Autodesk Inventor part; units mm, degrees
(part 4 of 4)
sketch "Sketch8" plane through (0, 0, 5) normal (0, 0, 1) x (1, 0, 0)
  line L0 (-35.5504, 47.4568) -> (35.8971, 47.4568) construction
  line L1 (35.8971, 47.4568) -> (35.8971, 30.428) construction
  line L2 (35.8971, 30.428) -> (-35.5504, 30.428) construction
  line L3 (-35.5504, 30.428) -> (-35.5504, 47.4568) construction
  line L4 (0.1734, 55.1961) -> (0.1734, 17.6773) construction
  line L5 (0, -39.5) -> (0, 79.5) construction
  spline S0 degree 2 poles (-22.5428, 39.6572) (-23.4481, 39.1897) (-24.7914, 39.1897) knots 0 0 0 1 1 1
  spline S1 degree 2 poles (-24.7914, 39.1897) (-26.5353, 39.1897) (-28.6281, 41.3863) (-28.6281, 43.1748) knots 0 0 0 1 2 2 2
  spline S2 degree 2 poles (-28.6281, 43.1748) (-28.6281, 45.0895) (-26.2682, 47.4568) (-24.4648, 47.4568) knots 0 0 0 1 2 2 2
  spline S3 degree 2 poles (-24.4648, 47.4568) (-23.3071, 47.4568) (-22.5428, 47.1303) knots 0 0 0 1 1 1
  line L6 (-22.5428, 47.1303) -> (-22.5428, 45.8093)
  spline S4 degree 2 poles (-22.5428, 45.8093) (-23.3517, 46.2917) (-24.3313, 46.2917) knots 0 0 0 1 1 1
  spline S5 degree 2 poles (-24.3313, 46.2917) (-25.63, 46.2917) (-27.2403, 44.6294) (-27.2403, 43.2416) knots 0 0 0 1 2 2 2
  spline S6 degree 2 poles (-27.2403, 43.2416) (-27.2403, 41.9132) (-25.7339, 40.3474) (-24.5094, 40.3474) knots 0 0 0 1 2 2 2
  spline S7 degree 2 poles (-24.5094, 40.3474) (-23.3739, 40.3474) (-22.5428, 40.8817) knots 0 0 0 1 1 1
  line L7 (-22.5428, 40.8817) -> (-22.5428, 39.6572)
  line L8 (-14.6021, 39.3232) -> (-15.9305, 39.3232)
  line L9 (-15.9305, 39.3232) -> (-15.9305, 42.7963)
  line L10 (-15.9305, 42.7963) -> (-19.7005, 42.7963)
  line L11 (-19.7005, 42.7963) -> (-19.7005, 39.3232)
  line L12 (-19.7005, 39.3232) -> (-21.0288, 39.3232)
  line L13 (-21.0288, 39.3232) -> (-21.0288, 47.3232)
  line L14 (-21.0288, 47.3232) -> (-19.7005, 47.3232)
  line L15 (-19.7005, 47.3232) -> (-19.7005, 43.9615)
  line L16 (-19.7005, 43.9615) -> (-15.9305, 43.9615)
  line L17 (-15.9305, 43.9615) -> (-15.9305, 47.3232)
  line L18 (-15.9305, 47.3232) -> (-14.6021, 47.3232)
  line L19 (-14.6021, 47.3232) -> (-14.6021, 39.3232)
  line L20 (-6.053, 39.3232) -> (-7.5075, 39.3232)
  line L21 (-7.5075, 39.3232) -> (-8.2274, 41.3566)
  line L22 (-8.2274, 41.3566) -> (-11.3739, 41.3566)
  line L23 (-11.3739, 41.3566) -> (-12.0715, 39.3232)
  line L24 (-12.0715, 39.3232) -> (-13.5186, 39.3232)
  line L25 (-13.5186, 39.3232) -> (-10.5205, 47.3232)
  line L26 (-10.5205, 47.3232) -> (-9.0288, 47.3232)
  line L27 (-9.0288, 47.3232) -> (-6.053, 39.3232)
  line L28 (-8.5836, 42.4401) -> (-9.6893, 45.6312)
  spline S8 degree 2 poles (-9.6893, 45.6312) (-9.7413, 45.7871) (-9.8006, 46.1359) knots 0 0 0 1 1 1
  line L29 (-9.8006, 46.1359) -> (-9.8229, 46.1359)
  spline S9 degree 2 poles (-9.8229, 46.1359) (-9.8674, 45.8168) (-9.9342, 45.6312) knots 0 0 0 1 1 1
  line L30 (-9.9342, 45.6312) -> (-11.0326, 42.4401)
  line L31 (-11.0326, 42.4401) -> (-8.5836, 42.4401)
  line L32 (-0.5242, 39.3232) -> (-4.9546, 39.3232)
  line L33 (-4.9546, 39.3232) -> (-4.9546, 47.3232)
  line L34 (-4.9546, 47.3232) -> (-3.6262, 47.3232)
  line L35 (-3.6262, 47.3232) -> (-3.6262, 40.4438)
  line L36 (-3.6262, 40.4438) -> (-0.5242, 40.4438)
  line L37 (-0.5242, 40.4438) -> (-0.5242, 39.3232)
  line L38 (9.2272, 39.3232) -> (7.9136, 39.3232)
  line L39 (7.9136, 39.3232) -> (7.9136, 44.5032)
  spline S10 degree 2 poles (7.9136, 44.5032) (7.9136, 45.134) (7.9879, 46.0542) knots 0 0 0 1 1 1
  line L40 (7.9879, 46.0542) -> (7.9656, 46.0542)
  spline S11 degree 2 poles (7.9656, 46.0542) (7.8469, 45.5348) (7.7504, 45.3047) knots 0 0 0 1 1 1
  line L41 (7.7504, 45.3047) -> (5.3608, 39.3232)
  line L42 (5.3608, 39.3232) -> (4.448, 39.3232)
  line L43 (4.448, 39.3232) -> (2.0509, 45.2602)
  spline S12 degree 2 poles (2.0509, 45.2602) (1.9545, 45.5199) (1.8431, 46.0542) knots 0 0 0 1 1 1
  line L44 (1.8431, 46.0542) -> (1.8209, 46.0542)
  spline S13 degree 2 poles (1.8209, 46.0542) (1.8654, 45.5793) (1.8654, 44.4884) knots 0 0 0 1 1 1
  line L45 (1.8654, 44.4884) -> (1.8654, 39.3232)
  line L46 (1.8654, 39.3232) -> (0.6335, 39.3232)
  line L47 (0.6335, 39.3232) -> (0.6335, 47.3232)
  line L48 (0.6335, 47.3232) -> (2.5036, 47.3232)
  line L49 (2.5036, 47.3232) -> (4.6038, 41.9949)
  spline S14 degree 2 poles (4.6038, 41.9949) (4.8487, 41.3789) (4.9229, 41.0821) knots 0 0 0 1 1 1
  line L50 (4.9229, 41.0821) -> (4.9452, 41.0821)
  spline S15 degree 2 poles (4.9452, 41.0821) (5.153, 41.7129) (5.2791, 42.0171) knots 0 0 0 1 1 1
  line L51 (5.2791, 42.0171) -> (7.4238, 47.3232)
  line L52 (7.4238, 47.3232) -> (9.2272, 47.3232)
  line L53 (9.2272, 47.3232) -> (9.2272, 39.3232)
  line L54 (15.6836, 39.3232) -> (11.1938, 39.3232)
  line L55 (11.1938, 39.3232) -> (11.1938, 47.3232)
  line L56 (11.1938, 47.3232) -> (15.5055, 47.3232)
  line L57 (15.5055, 47.3232) -> (15.5055, 46.1952)
  line L58 (15.5055, 46.1952) -> (12.5222, 46.1952)
  line L59 (12.5222, 46.1952) -> (12.5222, 43.9318)
  line L60 (12.5222, 43.9318) -> (15.2754, 43.9318)
  line L61 (15.2754, 43.9318) -> (15.2754, 42.8112)
  line L62 (15.2754, 42.8112) -> (12.5222, 42.8112)
  line L63 (12.5222, 42.8112) -> (12.5222, 40.4438)
  line L64 (12.5222, 40.4438) -> (15.6836, 40.4438)
  line L65 (15.6836, 40.4438) -> (15.6836, 39.3232)
  line L66 (23.2903, 39.3232) -> (21.7392, 39.3232)
  line L67 (21.7392, 39.3232) -> (20.4628, 41.468)
  spline S16 degree 2 poles (20.4628, 41.468) (20.2921, 41.7648) (19.9582, 42.1804) (19.6168, 42.4476) (19.2161, 42.5737) (18.9712, 42.5737) knots 0 0 0 1 2 3 4 4 4
  line L68 (18.9712, 42.5737) -> (18.4294, 42.5737)
  line L69 (18.4294, 42.5737) -> (18.4294, 39.3232)
  line L70 (18.4294, 39.3232) -> (17.1084, 39.3232)
  line L71 (17.1084, 39.3232) -> (17.1084, 47.3232)
  line L72 (17.1084, 47.3232) -> (19.743, 47.3232)
  spline S17 degree 2 poles (19.743, 47.3232) (20.307, 47.3232) (21.2569, 47.0561) (21.9619, 46.5143) (22.3552, 45.7054) (22.3552, 45.1637) knots 0 0 0 1 2 3 4 4 4
  spline S18 degree 2 poles (22.3552, 45.1637) (22.3552, 44.7407) (22.1029, 44.0357) (21.6428, 43.4791) (20.9897, 43.0932) (20.5815, 42.9893) knots 0 0 0 1 2 3 4 4 4
  line L73 (20.5815, 42.9893) -> (20.5815, 42.967)
  spline S19 degree 2 poles (20.5815, 42.967) (20.7968, 42.8409) (21.1233, 42.544) (21.4127, 42.2323) (21.6947, 41.839) (21.8728, 41.5719) knots 0 0 0 1 2 3 4 4 4
  line L74 (21.8728, 41.5719) -> (23.2903, 39.3232)
  line L75 (18.4294, 46.2472) -> (18.4294, 43.6498)
  line L76 (18.4294, 43.6498) -> (19.5352, 43.6498)
  spline S20 degree 2 poles (19.5352, 43.6498) (19.8469, 43.6498) (20.3589, 43.8427) (20.7448, 44.1989) (20.9526, 44.711) (20.9526, 45.0301) knots 0 0 0 1 2 3 4 4 4
  spline S21 degree 2 poles (20.9526, 45.0301) (20.9526, 45.6015) (20.2253, 46.2472) (19.55, 46.2472) knots 0 0 0 1 2 2 2
  line L77 (19.55, 46.2472) -> (18.4294, 46.2472)
  line L78 (23.8543, 39.6424) -> (23.8543, 41.0078)
  spline S22 degree 2 poles (23.8543, 41.0078) (24.0398, 40.8372) (24.5519, 40.57) (25.1159, 40.3919) (25.6873, 40.288) (25.9248, 40.288) knots 0 0 0 1 2 3 4 4 4
  spline S23 degree 2 poles (25.9248, 40.288) (26.7634, 40.288) (27.5871, 40.8446) (27.5871, 41.3789) knots 0 0 0 1 2 2 2
  spline S24 degree 2 poles (27.5871, 41.3789) (27.5871, 41.6609) (27.3125, 42.0765) (26.8227, 42.4253) (26.1548, 42.7444) (25.7764, 42.9151) knots 0 0 0 1 2 3 4 4 4
  spline S25 degree 2 poles (25.7764, 42.9151) (25.3682, 43.1303) (24.6706, 43.583) (24.1511, 44.1173) (23.8543, 44.8001) (23.8543, 45.2602) knots 0 0 0 1 2 3 4 4 4
  spline S26 degree 2 poles (23.8543, 45.2602) (23.8543, 45.8242) (24.3589, 46.6553) (25.1901, 47.1971) (26.2513, 47.4568) (26.8079, 47.4568) knots 0 0 0 1 2 3 4 4 4
  spline S27 degree 2 poles (26.8079, 47.4568) (28.0621, 47.4568) (28.6335, 47.1748) knots 0 0 0 1 1 1
  line L79 (28.6335, 47.1748) -> (28.6335, 45.8613)
  spline S28 degree 2 poles (28.6335, 45.8613) (27.9507, 46.3511) (26.8821, 46.3511) knots 0 0 0 1 1 1
  spline S29 degree 2 poles (26.8821, 46.3511) (26.5853, 46.3511) (25.999, 46.2398) (25.5389, 45.98) (25.2494, 45.5793) (25.2494, 45.2973) knots 0 0 0 1 2 3 4 4 4
  spline S30 degree 2 poles (25.2494, 45.2973) (25.2494, 45.0301) (25.4721, 44.6368) (25.9025, 44.3177) (26.5185, 44.006) (26.9266, 43.8279) knots 0 0 0 1 2 3 4 4 4
  spline S31 degree 2 poles (26.9266, 43.8279) (27.3422, 43.6127) (28.0843, 43.1303) (28.6483, 42.5514) (28.9823, 41.8464) (28.9823, 41.3937) knots 0 0 0 1 2 3 4 4 4
  spline S32 degree 2 poles (28.9823, 41.3937) (28.9823, 40.7852) (28.4925, 39.9466) (27.6613, 39.4271) (26.5778, 39.1897) (25.9693, 39.1897) knots 0 0 0 1 2 3 4 4 4
  spline S33 degree 2 poles (25.9693, 39.1897) (25.7689, 39.1897) (25.1827, 39.249) (24.5741, 39.3678) (24.025, 39.5385) (23.8543, 39.6424) knots 0 0 0 1 2 3 4 4 4
  line L80 (-23.3851, 31.9735) -> (-26.257, 23.9735)
  line L81 (-26.257, 23.9735) -> (-27.7413, 23.9735)
  line L82 (-27.7413, 23.9735) -> (-30.5613, 31.9735)
  line L83 (-30.5613, 31.9735) -> (-29.1142, 31.9735)
  line L84 (-29.1142, 31.9735) -> (-27.1402, 25.903)
  spline S34 degree 2 poles (-27.1402, 25.903) (-27.0437, 25.6136) (-26.9917, 25.2277) knots 0 0 0 1 1 1
  line L85 (-26.9917, 25.2277) -> (-26.9695, 25.2277)
  spline S35 degree 2 poles (-26.9695, 25.2277) (-26.9324, 25.5468) (-26.8062, 25.9179) knots 0 0 0 1 1 1
  line L86 (-26.8062, 25.9179) -> (-24.7877, 31.9735)
  line L87 (-24.7877, 31.9735) -> (-23.3851, 31.9735)
  line L88 (-17.834, 23.9735) -> (-22.3238, 23.9735)
  line L89 (-22.3238, 23.9735) -> (-22.3238, 31.9735)
  line L90 (-22.3238, 31.9735) -> (-18.0121, 31.9735)
  line L91 (-18.0121, 31.9735) -> (-18.0121, 30.8455)
  line L92 (-18.0121, 30.8455) -> (-20.9954, 30.8455)
  line L93 (-20.9954, 30.8455) -> (-20.9954, 28.582)
  line L94 (-20.9954, 28.582) -> (-18.2422, 28.582)
  line L95 (-18.2422, 28.582) -> (-18.2422, 27.4614)
  line L96 (-18.2422, 27.4614) -> (-20.9954, 27.4614)
  line L97 (-20.9954, 27.4614) -> (-20.9954, 25.0941)
  line L98 (-20.9954, 25.0941) -> (-17.834, 25.0941)
  line L99 (-17.834, 25.0941) -> (-17.834, 23.9735)
  line L100 (-10.2274, 23.9735) -> (-11.7784, 23.9735)
  line L101 (-11.7784, 23.9735) -> (-13.0548, 26.1182)
  spline S36 degree 2 poles (-13.0548, 26.1182) (-13.2255, 26.4151) (-13.5595, 26.8307) (-13.9008, 27.0978) (-14.3016, 27.224) (-14.5465, 27.224) knots 0 0 0 1 2 3 4 4 4
  line L102 (-14.5465, 27.224) -> (-15.0882, 27.224)
  line L103 (-15.0882, 27.224) -> (-15.0882, 23.9735)
  line L104 (-15.0882, 23.9735) -> (-16.4092, 23.9735)
  line L105 (-16.4092, 23.9735) -> (-16.4092, 31.9735)
  line L106 (-16.4092, 31.9735) -> (-13.7747, 31.9735)
  spline S37 degree 2 poles (-13.7747, 31.9735) (-13.2107, 31.9735) (-12.2608, 31.7063) (-11.5557, 31.1646) (-11.1624, 30.3557) (-11.1624, 29.814) knots 0 0 0 1 2 3 4 4 4
  spline S38 degree 2 poles (-11.1624, 29.814) (-11.1624, 29.3909) (-11.4147, 28.6859) (-11.8749, 28.1294) (-12.5279, 27.7435) (-12.9361, 27.6396) knots 0 0 0 1 2 3 4 4 4
  line L107 (-12.9361, 27.6396) -> (-12.9361, 27.6173)
  spline S39 degree 2 poles (-12.9361, 27.6173) (-12.7209, 27.4911) (-12.3943, 27.1943) (-12.1049, 26.8826) (-11.8229, 26.4893) (-11.6448, 26.2221) knots 0 0 0 1 2 3 4 4 4
  line L108 (-11.6448, 26.2221) -> (-10.2274, 23.9735)
  line L109 (-15.0882, 30.8974) -> (-15.0882, 28.3)
  line L110 (-15.0882, 28.3) -> (-13.9825, 28.3)
  spline S40 degree 2 poles (-13.9825, 28.3) (-13.6708, 28.3) (-13.1587, 28.493) (-12.7728, 28.8492) (-12.565, 29.3613) (-12.565, 29.6804) knots 0 0 0 1 2 3 4 4 4
  spline S41 degree 2 poles (-12.565, 29.6804) (-12.565, 30.2518) (-13.2923, 30.8974) (-13.9676, 30.8974) knots 0 0 0 1 2 2 2
  line L111 (-13.9676, 30.8974) -> (-15.0882, 30.8974)
  line L112 (-2.7172, 23.9735) -> (-4.1717, 23.9735)
  line L113 (-4.1717, 23.9735) -> (-4.8916, 26.0069)
  line L114 (-4.8916, 26.0069) -> (-8.0381, 26.0069)
  line L115 (-8.0381, 26.0069) -> (-8.7357, 23.9735)
  line L116 (-8.7357, 23.9735) -> (-10.1828, 23.9735)
  line L117 (-10.1828, 23.9735) -> (-7.1847, 31.9735)
  line L118 (-7.1847, 31.9735) -> (-5.693, 31.9735)
  line L119 (-5.693, 31.9735) -> (-2.7172, 23.9735)
  line L120 (-5.2478, 27.0904) -> (-6.3535, 30.2815)
  spline S42 degree 2 poles (-6.3535, 30.2815) (-6.4055, 30.4373) (-6.4648, 30.7861) knots 0 0 0 1 1 1
  line L121 (-6.4648, 30.7861) -> (-6.4871, 30.7861)
  spline S43 degree 2 poles (-6.4871, 30.7861) (-6.5316, 30.467) (-6.5984, 30.2815) knots 0 0 0 1 1 1
  line L122 (-6.5984, 30.2815) -> (-7.6967, 27.0904)
  line L123 (-7.6967, 27.0904) -> (-5.2478, 27.0904)
  line L124 (6.6558, 30.8455) -> (4.3552, 30.8455)
  line L125 (4.3552, 30.8455) -> (4.3552, 23.9735)
  line L126 (4.3552, 23.9735) -> (3.0268, 23.9735)
  line L127 (3.0268, 23.9735) -> (3.0268, 30.8455)
  line L128 (3.0268, 30.8455) -> (0.7337, 30.8455)
  line L129 (0.7337, 30.8455) -> (0.7337, 31.9735)
  line L130 (0.7337, 31.9735) -> (6.6558, 31.9735)
  line L131 (6.6558, 31.9735) -> (6.6558, 30.8455)
  line L132 (12.3181, 23.9735) -> (7.8283, 23.9735)
  line L133 (7.8283, 23.9735) -> (7.8283, 31.9735)
  line L134 (7.8283, 31.9735) -> (12.14, 31.9735)
  line L135 (12.14, 31.9735) -> (12.14, 30.8455)
  line L136 (12.14, 30.8455) -> (9.1567, 30.8455)
  line L137 (9.1567, 30.8455) -> (9.1567, 28.582)
  line L138 (9.1567, 28.582) -> (11.9099, 28.582)
  line L139 (11.9099, 28.582) -> (11.9099, 27.4614)
  line L140 (11.9099, 27.4614) -> (9.1567, 27.4614)
  line L141 (9.1567, 27.4614) -> (9.1567, 25.0941)
  line L142 (9.1567, 25.0941) -> (12.3181, 25.0941)
  line L143 (12.3181, 25.0941) -> (12.3181, 23.9735)
  line L144 (20.3181, 23.9735) -> (18.8636, 23.9735)
  line L145 (18.8636, 23.9735) -> (18.1437, 26.0069)
  line L146 (18.1437, 26.0069) -> (14.9971, 26.0069)
  line L147 (14.9971, 26.0069) -> (14.2995, 23.9735)
  line L148 (14.2995, 23.9735) -> (12.8524, 23.9735)
  line L149 (12.8524, 23.9735) -> (15.8506, 31.9735)
  line L150 (15.8506, 31.9735) -> (17.3422, 31.9735)
  line L151 (17.3422, 31.9735) -> (20.3181, 23.9735)
  line L152 (17.7875, 27.0904) -> (16.6817, 30.2815)
  spline S44 degree 2 poles (16.6817, 30.2815) (16.6298, 30.4373) (16.5704, 30.7861) knots 0 0 0 1 1 1
  line L153 (16.5704, 30.7861) -> (16.5482, 30.7861)
  spline S45 degree 2 poles (16.5482, 30.7861) (16.5036, 30.467) (16.4368, 30.2815) knots 0 0 0 1 1 1
  line L154 (16.4368, 30.2815) -> (15.3385, 27.0904)
  line L155 (15.3385, 27.0904) -> (17.7875, 27.0904)
  line L156 (30.0101, 23.9735) -> (28.6966, 23.9735)
  line L157 (28.6966, 23.9735) -> (28.6966, 29.1535)
  spline S46 degree 2 poles (28.6966, 29.1535) (28.6966, 29.7843) (28.7708, 30.7045) knots 0 0 0 1 1 1
  line L158 (28.7708, 30.7045) -> (28.7485, 30.7045)
  spline S47 degree 2 poles (28.7485, 30.7045) (28.6298, 30.185) (28.5333, 29.955) knots 0 0 0 1 1 1
  line L159 (28.5333, 29.955) -> (26.1437, 23.9735)
  line L160 (26.1437, 23.9735) -> (25.2309, 23.9735)
  line L161 (25.2309, 23.9735) -> (22.8339, 29.9104)
  spline S48 degree 2 poles (22.8339, 29.9104) (22.7374, 30.1702) (22.6261, 30.7045) knots 0 0 0 1 1 1
  line L162 (22.6261, 30.7045) -> (22.6038, 30.7045)
  spline S49 degree 2 poles (22.6038, 30.7045) (22.6483, 30.2295) (22.6483, 29.1386) knots 0 0 0 1 1 1
  line L163 (22.6483, 29.1386) -> (22.6483, 23.9735)
  line L164 (22.6483, 23.9735) -> (21.4164, 23.9735)
  line L165 (21.4164, 23.9735) -> (21.4164, 31.9735)
  line L166 (21.4164, 31.9735) -> (23.2866, 31.9735)
  line L167 (23.2866, 31.9735) -> (25.3867, 26.6451)
  spline S50 degree 2 poles (25.3867, 26.6451) (25.6316, 26.0292) (25.7059, 25.7323) knots 0 0 0 1 1 1
  line L168 (25.7059, 25.7323) -> (25.7281, 25.7323)
  spline S51 degree 2 poles (25.7281, 25.7323) (25.9359, 26.3631) (26.0621, 26.6674) knots 0 0 0 1 1 1
  line L169 (26.0621, 26.6674) -> (28.2068, 31.9735)
  line L170 (28.2068, 31.9735) -> (30.0101, 31.9735)
  line L171 (30.0101, 31.9735) -> (30.0101, 23.9735)
  spline S52 degree 2 poles (-22.5428, 39.6572) (-23.4481, 39.1897) (-24.7914, 39.1897) knots 0 0 0 1 1 1
  spline S53 degree 2 poles (-24.7914, 39.1897) (-26.5353, 39.1897) (-28.6281, 41.3863) (-28.6281, 43.1748) knots 0 0 0 1 2 2 2
  spline S54 degree 2 poles (-28.6281, 43.1748) (-28.6281, 45.0895) (-26.2682, 47.4568) (-24.4648, 47.4568) knots 0 0 0 1 2 2 2
  spline S55 degree 2 poles (-24.4648, 47.4568) (-23.3071, 47.4568) (-22.5428, 47.1303) knots 0 0 0 1 1 1
  line L172 (-22.5428, 47.1303) -> (-22.5428, 45.8093)
  spline S56 degree 2 poles (-22.5428, 45.8093) (-23.3517, 46.2917) (-24.3313, 46.2917) knots 0 0 0 1 1 1
  spline S57 degree 2 poles (-24.3313, 46.2917) (-25.63, 46.2917) (-27.2403, 44.6294) (-27.2403, 43.2416) knots 0 0 0 1 2 2 2
  spline S58 degree 2 poles (-27.2403, 43.2416) (-27.2403, 41.9132) (-25.7339, 40.3474) (-24.5094, 40.3474) knots 0 0 0 1 2 2 2
  spline S59 degree 2 poles (-24.5094, 40.3474) (-23.3739, 40.3474) (-22.5428, 40.8817) knots 0 0 0 1 1 1
  line L173 (-22.5428, 40.8817) -> (-22.5428, 39.6572)
  line L174 (-14.6021, 39.3232) -> (-15.9305, 39.3232)
  line L175 (-15.9305, 39.3232) -> (-15.9305, 42.7963)
  line L176 (-15.9305, 42.7963) -> (-19.7005, 42.7963)
  line L177 (-19.7005, 42.7963) -> (-19.7005, 39.3232)
  line L178 (-19.7005, 39.3232) -> (-21.0288, 39.3232)
  line L179 (-21.0288, 39.3232) -> (-21.0288, 47.3232)
  line L180 (-21.0288, 47.3232) -> (-19.7005, 47.3232)
  line L181 (-19.7005, 47.3232) -> (-19.7005, 43.9615)
  line L182 (-19.7005, 43.9615) -> (-15.9305, 43.9615)
  line L183 (-15.9305, 43.9615) -> (-15.9305, 47.3232)
  line L184 (-15.9305, 47.3232) -> (-14.6021, 47.3232)
  line L185 (-14.6021, 47.3232) -> (-14.6021, 39.3232)
  line L186 (-6.053, 39.3232) -> (-7.5075, 39.3232)
  line L187 (-7.5075, 39.3232) -> (-8.2274, 41.3566)
  line L188 (-8.2274, 41.3566) -> (-11.3739, 41.3566)
  line L189 (-11.3739, 41.3566) -> (-12.0715, 39.3232)
  line L190 (-12.0715, 39.3232) -> (-13.5186, 39.3232)
  line L191 (-13.5186, 39.3232) -> (-10.5205, 47.3232)
  line L192 (-10.5205, 47.3232) -> (-9.0288, 47.3232)
  line L193 (-9.0288, 47.3232) -> (-6.053, 39.3232)
  line L194 (-8.5836, 42.4401) -> (-9.6893, 45.6312)
  spline S60 degree 2 poles (-9.6893, 45.6312) (-9.7413, 45.7871) (-9.8006, 46.1359) knots 0 0 0 1 1 1
  line L195 (-9.8006, 46.1359) -> (-9.8229, 46.1359)
  spline S61 degree 2 poles (-9.8229, 46.1359) (-9.8674, 45.8168) (-9.9342, 45.6312) knots 0 0 0 1 1 1
  line L196 (-9.9342, 45.6312) -> (-11.0326, 42.4401)
  line L197 (-11.0326, 42.4401) -> (-8.5836, 42.4401)
  line L198 (-0.5242, 39.3232) -> (-4.9546, 39.3232)
  line L199 (-4.9546, 39.3232) -> (-4.9546, 47.3232)
  line L200 (-4.9546, 47.3232) -> (-3.6262, 47.3232)
  line L201 (-3.6262, 47.3232) -> (-3.6262, 40.4438)
  line L202 (-3.6262, 40.4438) -> (-0.5242, 40.4438)
  line L203 (-0.5242, 40.4438) -> (-0.5242, 39.3232)
  line L204 (9.2272, 39.3232) -> (7.9136, 39.3232)
  line L205 (7.9136, 39.3232) -> (7.9136, 44.5032)
  spline S62 degree 2 poles (7.9136, 44.5032) (7.9136, 45.134) (7.9879, 46.0542) knots 0 0 0 1 1 1
  line L206 (7.9879, 46.0542) -> (7.9656, 46.0542)
  spline S63 degree 2 poles (7.9656, 46.0542) (7.8469, 45.5348) (7.7504, 45.3047) knots 0 0 0 1 1 1
  line L207 (7.7504, 45.3047) -> (5.3608, 39.3232)
  line L208 (5.3608, 39.3232) -> (4.448, 39.3232)
  line L209 (4.448, 39.3232) -> (2.0509, 45.2602)
  spline S64 degree 2 poles (2.0509, 45.2602) (1.9545, 45.5199) (1.8431, 46.0542) knots 0 0 0 1 1 1
  line L210 (1.8431, 46.0542) -> (1.8209, 46.0542)
  spline S65 degree 2 poles (1.8209, 46.0542) (1.8654, 45.5793) (1.8654, 44.4884) knots 0 0 0 1 1 1
  line L211 (1.8654, 44.4884) -> (1.8654, 39.3232)
  line L212 (1.8654, 39.3232) -> (0.6335, 39.3232)
  line L213 (0.6335, 39.3232) -> (0.6335, 47.3232)
  line L214 (0.6335, 47.3232) -> (2.5036, 47.3232)
  line L215 (2.5036, 47.3232) -> (4.6038, 41.9949)
  spline S66 degree 2 poles (4.6038, 41.9949) (4.8487, 41.3789) (4.9229, 41.0821) knots 0 0 0 1 1 1
  line L216 (4.9229, 41.0821) -> (4.9452, 41.0821)
  spline S67 degree 2 poles (4.9452, 41.0821) (5.153, 41.7129) (5.2791, 42.0171) knots 0 0 0 1 1 1
  line L217 (5.2791, 42.0171) -> (7.4238, 47.3232)
  line L218 (7.4238, 47.3232) -> (9.2272, 47.3232)
  line L219 (9.2272, 47.3232) -> (9.2272, 39.3232)
  line L220 (15.6836, 39.3232) -> (11.1938, 39.3232)
  line L221 (11.1938, 39.3232) -> (11.1938, 47.3232)
  line L222 (11.1938, 47.3232) -> (15.5055, 47.3232)
  line L223 (15.5055, 47.3232) -> (15.5055, 46.1952)
  line L224 (15.5055, 46.1952) -> (12.5222, 46.1952)
  line L225 (12.5222, 46.1952) -> (12.5222, 43.9318)
  line L226 (12.5222, 43.9318) -> (15.2754, 43.9318)
  line L227 (15.2754, 43.9318) -> (15.2754, 42.8112)
  line L228 (15.2754, 42.8112) -> (12.5222, 42.8112)
  line L229 (12.5222, 42.8112) -> (12.5222, 40.4438)
  line L230 (12.5222, 40.4438) -> (15.6836, 40.4438)
  line L231 (15.6836, 40.4438) -> (15.6836, 39.3232)
  line L232 (23.2903, 39.3232) -> (21.7392, 39.3232)
  line L233 (21.7392, 39.3232) -> (20.4628, 41.468)
  spline S68 degree 2 poles (20.4628, 41.468) (20.2921, 41.7648) (19.9582, 42.1804) (19.6168, 42.4476) (19.2161, 42.5737) (18.9712, 42.5737) knots 0 0 0 1 2 3 4 4 4
  line L234 (18.9712, 42.5737) -> (18.4294, 42.5737)
  line L235 (18.4294, 42.5737) -> (18.4294, 39.3232)
  line L236 (18.4294, 39.3232) -> (17.1084, 39.3232)
  line L237 (17.1084, 39.3232) -> (17.1084, 47.3232)
  line L238 (17.1084, 47.3232) -> (19.743, 47.3232)
  spline S69 degree 2 poles (19.743, 47.3232) (20.307, 47.3232) (21.2569, 47.0561) (21.9619, 46.5143) (22.3552, 45.7054) (22.3552, 45.1637) knots 0 0 0 1 2 3 4 4 4
  spline S70 degree 2 poles (22.3552, 45.1637) (22.3552, 44.7407) (22.1029, 44.0357) (21.6428, 43.4791) (20.9897, 43.0932) (20.5815, 42.9893) knots 0 0 0 1 2 3 4 4 4
  line L239 (20.5815, 42.9893) -> (20.5815, 42.967)
  spline S71 degree 2 poles (20.5815, 42.967) (20.7968, 42.8409) (21.1233, 42.544) (21.4127, 42.2323) (21.6947, 41.839) (21.8728, 41.5719) knots 0 0 0 1 2 3 4 4 4
  line L240 (21.8728, 41.5719) -> (23.2903, 39.3232)
  line L241 (18.4294, 46.2472) -> (18.4294, 43.6498)
  line L242 (18.4294, 43.6498) -> (19.5352, 43.6498)
  spline S72 degree 2 poles (19.5352, 43.6498) (19.8469, 43.6498) (20.3589, 43.8427) (20.7448, 44.1989) (20.9526, 44.711) (20.9526, 45.0301) knots 0 0 0 1 2 3 4 4 4
  spline S73 degree 2 poles (20.9526, 45.0301) (20.9526, 45.6015) (20.2253, 46.2472) (19.55, 46.2472) knots 0 0 0 1 2 2 2
  line L243 (19.55, 46.2472) -> (18.4294, 46.2472)
  line L244 (23.8543, 39.6424) -> (23.8543, 41.0078)
  spline S74 degree 2 poles (23.8543, 41.0078) (24.0398, 40.8372) (24.5519, 40.57) (25.1159, 40.3919) (25.6873, 40.288) (25.9248, 40.288) knots 0 0 0 1 2 3 4 4 4
  spline S75 degree 2 poles (25.9248, 40.288) (26.7634, 40.288) (27.5871, 40.8446) (27.5871, 41.3789) knots 0 0 0 1 2 2 2
  spline S76 degree 2 poles (27.5871, 41.3789) (27.5871, 41.6609) (27.3125, 42.0765) (26.8227, 42.4253) (26.1548, 42.7444) (25.7764, 42.9151) knots 0 0 0 1 2 3 4 4 4
  spline S77 degree 2 poles (25.7764, 42.9151) (25.3682, 43.1303) (24.6706, 43.583) (24.1511, 44.1173) (23.8543, 44.8001) (23.8543, 45.2602) knots 0 0 0 1 2 3 4 4 4
  spline S78 degree 2 poles (23.8543, 45.2602) (23.8543, 45.8242) (24.3589, 46.6553) (25.1901, 47.1971) (26.2513, 47.4568) (26.8079, 47.4568) knots 0 0 0 1 2 3 4 4 4
  spline S79 degree 2 poles (26.8079, 47.4568) (28.0621, 47.4568) (28.6335, 47.1748) knots 0 0 0 1 1 1
  line L245 (28.6335, 47.1748) -> (28.6335, 45.8613)
  spline S80 degree 2 poles (28.6335, 45.8613) (27.9507, 46.3511) (26.8821, 46.3511) knots 0 0 0 1 1 1
  spline S81 degree 2 poles (26.8821, 46.3511) (26.5853, 46.3511) (25.999, 46.2398) (25.5389, 45.98) (25.2494, 45.5793) (25.2494, 45.2973) knots 0 0 0 1 2 3 4 4 4
  spline S82 degree 2 poles (25.2494, 45.2973) (25.2494, 45.0301) (25.4721, 44.6368) (25.9025, 44.3177) (26.5185, 44.006) (26.9266, 43.8279) knots 0 0 0 1 2 3 4 4 4
  spline S83 degree 2 poles (26.9266, 43.8279) (27.3422, 43.6127) (28.0843, 43.1303) (28.6483, 42.5514) (28.9823, 41.8464) (28.9823, 41.3937) knots 0 0 0 1 2 3 4 4 4
  spline S84 degree 2 poles (28.9823, 41.3937) (28.9823, 40.7852) (28.4925, 39.9466) (27.6613, 39.4271) (26.5778, 39.1897) (25.9693, 39.1897) knots 0 0 0 1 2 3 4 4 4
  spline S85 degree 2 poles (25.9693, 39.1897) (25.7689, 39.1897) (25.1827, 39.249) (24.5741, 39.3678) (24.025, 39.5385) (23.8543, 39.6424) knots 0 0 0 1 2 3 4 4 4
  line L246 (-23.3851, 31.9735) -> (-26.257, 23.9735)
  line L247 (-26.257, 23.9735) -> (-27.7413, 23.9735)
  line L248 (-27.7413, 23.9735) -> (-30.5613, 31.9735)
  line L249 (-30.5613, 31.9735) -> (-29.1142, 31.9735)
  line L250 (-29.1142, 31.9735) -> (-27.1402, 25.903)
  spline S86 degree 2 poles (-27.1402, 25.903) (-27.0437, 25.6136) (-26.9917, 25.2277) knots 0 0 0 1 1 1
  line L251 (-26.9917, 25.2277) -> (-26.9695, 25.2277)
  spline S87 degree 2 poles (-26.9695, 25.2277) (-26.9324, 25.5468) (-26.8062, 25.9179) knots 0 0 0 1 1 1
  line L252 (-26.8062, 25.9179) -> (-24.7877, 31.9735)
  line L253 (-24.7877, 31.9735) -> (-23.3851, 31.9735)
  line L254 (-17.834, 23.9735) -> (-22.3238, 23.9735)
  line L255 (-22.3238, 23.9735) -> (-22.3238, 31.9735)
  line L256 (-22.3238, 31.9735) -> (-18.0121, 31.9735)
  line L257 (-18.0121, 31.9735) -> (-18.0121, 30.8455)
  line L258 (-18.0121, 30.8455) -> (-20.9954, 30.8455)
  line L259 (-20.9954, 30.8455) -> (-20.9954, 28.582)
  line L260 (-20.9954, 28.582) -> (-18.2422, 28.582)
  line L261 (-18.2422, 28.582) -> (-18.2422, 27.4614)
  line L262 (-18.2422, 27.4614) -> (-20.9954, 27.4614)
  line L263 (-20.9954, 27.4614) -> (-20.9954, 25.0941)
  line L264 (-20.9954, 25.0941) -> (-17.834, 25.0941)
  line L265 (-17.834, 25.0941) -> (-17.834, 23.9735)
  line L266 (-10.2274, 23.9735) -> (-11.7784, 23.9735)
  line L267 (-11.7784, 23.9735) -> (-13.0548, 26.1182)
  spline S88 degree 2 poles (-13.0548, 26.1182) (-13.2255, 26.4151) (-13.5595, 26.8307) (-13.9008, 27.0978) (-14.3016, 27.224) (-14.5465, 27.224) knots 0 0 0 1 2 3 4 4 4
  line L268 (-14.5465, 27.224) -> (-15.0882, 27.224)
  line L269 (-15.0882, 27.224) -> (-15.0882, 23.9735)
  line L270 (-15.0882, 23.9735) -> (-16.4092, 23.9735)
  line L271 (-16.4092, 23.9735) -> (-16.4092, 31.9735)
  line L272 (-16.4092, 31.9735) -> (-13.7747, 31.9735)
  spline S89 degree 2 poles (-13.7747, 31.9735) (-13.2107, 31.9735) (-12.2608, 31.7063) (-11.5557, 31.1646) (-11.1624, 30.3557) (-11.1624, 29.814) knots 0 0 0 1 2 3 4 4 4
  spline S90 degree 2 poles (-11.1624, 29.814) (-11.1624, 29.3909) (-11.4147, 28.6859) (-11.8749, 28.1294) (-12.5279, 27.7435) (-12.9361, 27.6396) knots 0 0 0 1 2 3 4 4 4
  line L273 (-12.9361, 27.6396) -> (-12.9361, 27.6173)
  spline S91 degree 2 poles (-12.9361, 27.6173) (-12.7209, 27.4911) (-12.3943, 27.1943) (-12.1049, 26.8826) (-11.8229, 26.4893) (-11.6448, 26.2221) knots 0 0 0 1 2 3 4 4 4
  line L274 (-11.6448, 26.2221) -> (-10.2274, 23.9735)
  line L275 (-15.0882, 30.8974) -> (-15.0882, 28.3)
  line L276 (-15.0882, 28.3) -> (-13.9825, 28.3)
  spline S92 degree 2 poles (-13.9825, 28.3) (-13.6708, 28.3) (-13.1587, 28.493) (-12.7728, 28.8492) (-12.565, 29.3613) (-12.565, 29.6804) knots 0 0 0 1 2 3 4 4 4
  spline S93 degree 2 poles (-12.565, 29.6804) (-12.565, 30.2518) (-13.2923, 30.8974) (-13.9676, 30.8974) knots 0 0 0 1 2 2 2
  line L277 (-13.9676, 30.8974) -> (-15.0882, 30.8974)
  line L278 (-2.7172, 23.9735) -> (-4.1717, 23.9735)
  line L279 (-4.1717, 23.9735) -> (-4.8916, 26.0069)
  line L280 (-4.8916, 26.0069) -> (-8.0381, 26.0069)
  line L281 (-8.0381, 26.0069) -> (-8.7357, 23.9735)
  line L282 (-8.7357, 23.9735) -> (-10.1828, 23.9735)
  line L283 (-10.1828, 23.9735) -> (-7.1847, 31.9735)
  line L284 (-7.1847, 31.9735) -> (-5.693, 31.9735)
  line L285 (-5.693, 31.9735) -> (-2.7172, 23.9735)
  line L286 (-5.2478, 27.0904) -> (-6.3535, 30.2815)
  spline S94 degree 2 poles (-6.3535, 30.2815) (-6.4055, 30.4373) (-6.4648, 30.7861) knots 0 0 0 1 1 1
  line L287 (-6.4648, 30.7861) -> (-6.4871, 30.7861)
  spline S95 degree 2 poles (-6.4871, 30.7861) (-6.5316, 30.467) (-6.5984, 30.2815) knots 0 0 0 1 1 1
  line L288 (-6.5984, 30.2815) -> (-7.6967, 27.0904)
  line L289 (-7.6967, 27.0904) -> (-5.2478, 27.0904)
  line L290 (6.6558, 30.8455) -> (4.3552, 30.8455)
  line L291 (4.3552, 30.8455) -> (4.3552, 23.9735)
  line L292 (4.3552, 23.9735) -> (3.0268, 23.9735)
  line L293 (3.0268, 23.9735) -> (3.0268, 30.8455)
  line L294 (3.0268, 30.8455) -> (0.7337, 30.8455)
  line L295 (0.7337, 30.8455) -> (0.7337, 31.9735)
  line L296 (0.7337, 31.9735) -> (6.6558, 31.9735)
  line L297 (6.6558, 31.9735) -> (6.6558, 30.8455)
  line L298 (12.3181, 23.9735) -> (7.8283, 23.9735)
  line L299 (7.8283, 23.9735) -> (7.8283, 31.9735)
  line L300 (7.8283, 31.9735) -> (12.14, 31.9735)
  line L301 (12.14, 31.9735) -> (12.14, 30.8455)
  line L302 (12.14, 30.8455) -> (9.1567, 30.8455)
  line L303 (9.1567, 30.8455) -> (9.1567, 28.582)
  line L304 (9.1567, 28.582) -> (11.9099, 28.582)
  line L305 (11.9099, 28.582) -> (11.9099, 27.4614)
  line L306 (11.9099, 27.4614) -> (9.1567, 27.4614)
  line L307 (9.1567, 27.4614) -> (9.1567, 25.0941)
  line L308 (9.1567, 25.0941) -> (12.3181, 25.0941)
  line L309 (12.3181, 25.0941) -> (12.3181, 23.9735)
  line L310 (20.3181, 23.9735) -> (18.8636, 23.9735)
  line L311 (18.8636, 23.9735) -> (18.1437, 26.0069)
  line L312 (18.1437, 26.0069) -> (14.9971, 26.0069)
  line L313 (14.9971, 26.0069) -> (14.2995, 23.9735)
  line L314 (14.2995, 23.9735) -> (12.8524, 23.9735)
  line L315 (12.8524, 23.9735) -> (15.8506, 31.9735)
  line L316 (15.8506, 31.9735) -> (17.3422, 31.9735)
  line L317 (17.3422, 31.9735) -> (20.3181, 23.9735)
  line L318 (17.7875, 27.0904) -> (16.6817, 30.2815)
  spline S96 degree 2 poles (16.6817, 30.2815) (16.6298, 30.4373) (16.5704, 30.7861) knots 0 0 0 1 1 1
  line L319 (16.5704, 30.7861) -> (16.5482, 30.7861)
  spline S97 degree 2 poles (16.5482, 30.7861) (16.5036, 30.467) (16.4368, 30.2815) knots 0 0 0 1 1 1
  line L320 (16.4368, 30.2815) -> (15.3385, 27.0904)
  line L321 (15.3385, 27.0904) -> (17.7875, 27.0904)
  line L322 (30.0101, 23.9735) -> (28.6966, 23.9735)
  line L323 (28.6966, 23.9735) -> (28.6966, 29.1535)
  spline S98 degree 2 poles (28.6966, 29.1535) (28.6966, 29.7843) (28.7708, 30.7045) knots 0 0 0 1 1 1
  line L324 (28.7708, 30.7045) -> (28.7485, 30.7045)
  spline S99 degree 2 poles (28.7485, 30.7045) (28.6298, 30.185) (28.5333, 29.955) knots 0 0 0 1 1 1
  line L325 (28.5333, 29.955) -> (26.1437, 23.9735)
  line L326 (26.1437, 23.9735) -> (25.2309, 23.9735)
  line L327 (25.2309, 23.9735) -> (22.8339, 29.9104)
  spline S100 degree 2 poles (22.8339, 29.9104) (22.7374, 30.1702) (22.6261, 30.7045) knots 0 0 0 1 1 1
  line L328 (22.6261, 30.7045) -> (22.6038, 30.7045)
  spline S101 degree 2 poles (22.6038, 30.7045) (22.6483, 30.2295) (22.6483, 29.1386) knots 0 0 0 1 1 1
  line L329 (22.6483, 29.1386) -> (22.6483, 23.9735)
  line L330 (22.6483, 23.9735) -> (21.4164, 23.9735)
  line L331 (21.4164, 23.9735) -> (21.4164, 31.9735)
  line L332 (21.4164, 31.9735) -> (23.2866, 31.9735)
  line L333 (23.2866, 31.9735) -> (25.3867, 26.6451)
  spline S102 degree 2 poles (25.3867, 26.6451) (25.6316, 26.0292) (25.7059, 25.7323) knots 0 0 0 1 1 1
  line L334 (25.7059, 25.7323) -> (25.7281, 25.7323)
  spline S103 degree 2 poles (25.7281, 25.7323) (25.9359, 26.3631) (26.0621, 26.6674) knots 0 0 0 1 1 1
  line L335 (26.0621, 26.6674) -> (28.2068, 31.9735)
  line L336 (28.2068, 31.9735) -> (30.0101, 31.9735)
  line L337 (30.0101, 31.9735) -> (30.0101, 23.9735)
  point P0 (0, 0)
  constraints: 2 end point, 1 vertical, 3 other
extrude "Extrusion6" cut sketch "Sketch8" against normal blind 1
extrude "Extrusion7" add sketch "Sketch8" against normal up to next separate body
equation "\"d5\" = mountingScrewSize"
equation "\"d6\" = d5"
equation "\"d18\" = d6"
equation "\"d21\" = d20"
equation "\"d22\" = d20"
equation "\"d23\" = d20"
equation "\"d36\" = mountingScrewSize"
equation "\"mountingScrewSize\" = 3"
body "Solid1"
body "Solid2"
